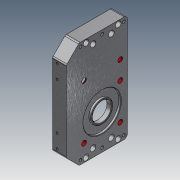
# Autodesk Inventor part: J008101
Saved by Autodesk Inventor 2018.3 (Build 223284000, 284)
## iProperties
Created: 2014-12-15
Material: ALUMINUM, 6061-T651
Vendor: HHMI: JFRC - ID&F
Document SubType Name: Modeling
Designer: ARNOLDJ
Density: 2.7 g/cm^3
Mass: 248.908 g
Surface Area: 451.626 cm^2
Volume: 92.1883 cm^3
Part Number: J008101
Description: BBP OUTER POSARM
Project: COMMON
Appearance: Polished Brushed
RuleStatus: InUse
AfterDocSave0: file://Part Number Cleaner
LAB/DEPT: COMMON
REQUESTING SCIENTIST: COMMON
SURFACE ROUGHNESS: 63 Ra
DESIGN DEPARTMENT: HHMI: JRC - ID&F
SPECIAL FINISH: ANODIZE PER MIL-A-8625F, TYPE II, CLASS 2 (BLACK)
ALTERED ITEM PART NUMBER: N/A
ALTERED ITEM VENDOR: N/A
ALTERED ITEM DESCRIPTION: N/A
Revision Number: -
Autodesk Inventor part; units mm, degrees
sketch "Sketch1" plane through (0, 0, 0) normal (0, 0, 1) x (1, 0, 0)
  line L0 (0, 127.7214) -> (0, -77.7088) projected
  line L1 (-22.86, 0) -> (3.81, 0) projected
  line L2 (-19.05, -48.3616) -> (-19.05, 98.3742)
  line L3 (0, -48.3616) -> (0, 98.3742)
  line L4 (-19.05, 98.3742) -> (0, 98.3742)
  line L5 (0, -48.3616) -> (-19.05, -48.3616)
  line L6 (-9.525, 98.3742) -> (-9.525, -48.3616) construction
  point P0 (0, 0)
  dimension "d5" = 19.05
  dimension "d67" = 0
  dimension "d149" = 48.3616
  dimension "d150" = 98.3742
  constraints: 10 end point, 2 horizontal, 2 midpoint, 1 perpendicular, 1 vertical
  measures "d5" distance between parallel lines of L2 L3
  measures "d67" distance between parallel lines of L0 L3
  measures "d149" distance between parallel lines of L5 L1
  measures "d150" distance between parallel lines of L1 L4
extrude "Extrusion1" add sketch "Sketch1" along normal blind 49.53 and the other way blind 34.925
sketch "Sketch6" plane through (0, 0, 0) normal (1, 0, 0) x (0, 1, 0)
  line L0 (0, 40.7695) -> (0, -40.1472) projected
  line L1 (-50.1548, 0) -> (123.129, 0) projected
  line L2 (-25, 25) -> (25, 25)
  line L3 (25, 25) -> (25, -25)
  line L4 (25, -25) -> (-25, -25)
  line L5 (-25, -25) -> (-25, 25)
  line L6 (0, 25) -> (0, -25) construction
  line L7 (-25, 0) -> (25, 0) construction
  point P0 (0, 0)
  point P1 (50, 25)
  point P2 (50, -25)
  dimension "d49" = 50
  dimension "d50" = 50
  dimension "d51" = 0
  dimension "d52" = 0
  dimension "d388" = 25
  constraints: 12 end point, 4 coincident, 4 midpoint, 2 parallel, 1 horizontal, 1 horizontal alignment, 1 perpendicular, 1 vertical alignment
  measures "d49" distance of L2.start L2.end
  measures "d50" distance of L4.end L2.start
  measures "d51" distance between parallel lines of L0 L6
  measures "d52" distance between parallel lines of L1 L7
  measures "d388" distance from line of L3 point (50, 25)
hole "Hole3" at (0, -25, 25) at (0, 25, -25) at (0, -25, -25) direction (-1, 0, 0) diameter 6.7564 end through all clearance for "Socket Head Cap Screw" size "M6" standard "Ansi Metric M Profile"
sketch "Sketch9" plane through (-19.05, -48.3616, 49.53) normal (-1, 0, 0) x (0, 0, 1)
  circle A0 centre (-49.53, 48.3616) radius 30 construction
  line L0 (-84.455, 146.7358) -> (-84.455, 0) projected
  line L1 (0, 0) -> (0, 146.7358) projected
  circle A1 centre (-49.53, 48.3616) radius 31.0125 construction
  line L2 (-84.455, 0) -> (0, 0) projected
  line L3 (-80.5425, 79.3741) -> (-16.0265, 79.3741)
  line L4 (-16.0265, 79.3741) -> (-16.0265, 16.5091)
  line L5 (-16.0265, 16.5091) -> (-80.5425, 16.5091)
  line L6 (-80.5425, 16.5091) -> (-80.5425, 79.3741)
  line L7 (-80.5425, 79.3741) -> (-16.0265, 79.3741)
  dimension "d80" = 60
  dimension "d87" = 62.025
  dimension "d174" = 62.865
  dimension "d231" = 64.516
  constraints: 10 end point, 2 centre point, 2 coincident, 2 horizontal, 2 parallel, 2 tangent, 1 perpendicular
  measures "d80" diameter of A0
  measures "d87" diameter of A1
  measures "d174" distance of L5.end L3.start
  measures "d231" distance between parallel lines of L4 L6
ref_plane "Work Plane1" through (-19.05, 0, 0) normal (1, 0, 0) x (0, 1, 0)
extrude "Extrusion5-Motor Cutout" cut sketch "Sketch9" against normal blind 12.7
sketch "Sketch20" plane through (-19.05, -48.3616, 49.53) normal (-1, 0, 0) x (0, 0, 1)
  line L0 (-80.5425, 16.5091) -> (-80.5425, 79.3741) projected
  line L1 (-16.0265, 16.5091) -> (-80.5425, 16.5091) projected
  line L2 (-16.0265, 79.3741) -> (-16.0265, 16.5091) projected
  line L3 (-79.2725, 129.5908) -> (-4.445, 129.5908)
  line L4 (-4.445, 129.5908) -> (-4.445, 16.5091)
  line L5 (-4.445, 16.5091) -> (-79.2725, 16.5091)
  line L6 (-79.2725, 16.5091) -> (-79.2725, 129.5908)
  line L7 (-80.5425, 79.3741) -> (-16.0265, 79.3741) projected
  line L8 (0, 0) -> (0, 146.7358) projected
  line L9 (-84.455, 146.7358) -> (-84.455, 0) projected
  line L10 (0, 146.7358) -> (-84.455, 146.7358) projected
  point P0 (-49.53, 48.3616)
  dimension "d185" = 64.516
  dimension "d232" = 4.445
  dimension "d233" = 3.9125
  dimension "d246" = 17.145
  dimension "d334" = 0
  constraints: 8 end point, 2 parallel, 1 horizontal, 1 perpendicular
  measures "d185" distance of L0.end L2.start
  measures "d232" distance between parallel lines of L8 L4
  measures "d233" distance between parallel lines of L0 L9
  measures "d246" distance between parallel lines of L10 L3
  measures "d334" distance between parallel lines of L5 L1
extrude "Extrusion12-Complete the Box cutout" cut sketch "Sketch20" against normal blind 11.43 contours L6 L7 L2 L1 | L6 L3 L4 L5 L2 L7
sketch "Sketch10" plane through (0, 0, 0) normal (1, 0, 0) x (0, 1, 0)
  circle A0 centre (0, 0) radius 13
  dimension "d93" = 26
  constraints: 1 centre point, 1 coincident
  measures "d93" diameter of A0
extrude "Extrusion6" cut sketch "Sketch10" against normal blind 25.4
sketch "Sketch25" plane through (-7.62, -48.3616, 49.53) normal (-1, 0, 0) x (0, 0, 1)
  line L0 (-4.445, 129.5908) -> (-4.445, 16.5091) projected
  line L1 (-79.2725, 129.5908) -> (-4.445, 129.5908) projected
  line L2 (-79.2725, 79.3741) -> (-79.2725, 129.5908) projected
  line L3 (-4.445, 129.5908) -> (-40.6387, 129.5908)
  line L4 (-40.6387, 84.4541) -> (-4.445, 84.4541)
  line L5 (-4.445, 84.4541) -> (-4.445, 129.5908)
  line L6 (-4.445, 129.5908) -> (-69.1125, 129.5908)
  line L7 (-69.1125, 129.5908) -> (-69.1125, 84.4541)
  line L8 (-69.1125, 84.4541) -> (-4.445, 84.4541)
  line L9 (-16.0265, 79.3741) -> (-79.2725, 79.3741) projected
  line L10 (-16.0265, 16.5091) -> (-4.445, 16.5091) projected
  line L11 (-4.445, 79.3741) -> (-13.4865, 79.3741)
  line L12 (-13.4865, 79.3741) -> (-13.4865, 16.5091)
  line L13 (-13.4865, 16.5091) -> (-4.445, 16.5091)
  line L14 (-4.445, 16.5091) -> (-4.445, 79.3741)
  point P0 (-49.53, 48.3616)
  dimension "d248" = 0
  dimension "d249" = 5.08
  dimension "d250" = 0
  dimension "d252" = 10.16
  dimension "d356" = 0
  dimension "d357" = 2.54
  constraints: 20 end point, 4 parallel, 3 horizontal, 2 perpendicular, 2 point on line
  measures "d248" distance between parallel lines of L1 L3
  measures "d249" distance between parallel lines of L4 L9
  measures "d250" distance between parallel lines of L5 L0
  measures "d252" distance between parallel lines of L7 L2
  measures "d356" distance between parallel lines of L14 L0
  measures "d357" distance from line of L9.start L12
extrude "Extrusion16" cut sketch "Sketch25" against normal blind 3.81
fillet "Fillet17" radius 3.175 7 edges at (-5.715, 36.0925, -19.5825) (-5.715, 36.0925, 45.085) (-5.715, 81.2292, -19.5825) (-5.715, 31.0125, 45.085) (-5.715, 31.0125, 36.0435) (-5.715, -31.8525, 36.0435) (-11.43, -31.8525, 45.085)
fillet "Fillet23" radius 1.651 1 edges at (-11.43, 81.2292, 45.085)
chamfer "Chamfer5" distance 17.78 angle 45 1 edges at (-9.525, -48.3616, 49.53)
chamfer "Chamfer8" distance 3.175 angle 45 2 edges at (-9.525, 98.3742, -34.925) (-9.525, -48.3616, -34.925)
chamfer "Chamfer9" distance 17.78 angle 45 1 edges at (-9.525, 98.3742, 49.53)
sketch "Sketch22" plane through (0, 0, 0) normal (1, 0, 0) x (0, 1, 0)
  point P0 (0, 0)
sketch "Sketch23" plane through (0, -31.8516, -34.925) normal (1, 0, 0) x (0, 0, -1)
  circle A0 centre (-34.925, 31.8516) radius 15.24
  circle A1 centre (-34.925, 31.8516) radius 26.035
  dimension "d221" = 52.07
  dimension "d222" = 30.48
  constraints: 2 centre point, 2 coincident
  measures "d221" diameter of A1
  measures "d222" diameter of A0
extrude "Extrusion14-rear circ cutout" cut sketch "Sketch23" against normal blind 3.175
chamfer "Chamfer10 Around rear circular cutout" distance 0.635 angle 45 3 edges at (0, 0, 26.035) (0, 0, 15.24) (0, -13, 0)
fillet "Fillet22" radius 2.413 1 edges at (-12.7, 31.0125, -31.0125)
sketch "Sketch24" plane through (-19.05, 0, 0) normal (1, 0, 0) x (0, 1, 0)
  line L0 (98.3742, 31.75) -> (98.3742, -31.75) projected
  line L1 (31.0125, -29.7425) -> (81.2292, -29.7425) projected
  line L2 (62.6618, -29.7425) -> (27.7368, -29.7425)
  line L3 (27.7368, -29.7425) -> (27.7368, -31.6475)
  line L4 (27.7368, -31.6475) -> (62.6618, -31.6475)
  line L5 (62.6618, -31.6475) -> (62.6618, -29.7425)
  point P0 (0, 0)
  point P1 (106.426, 30.4349)
  point P2 (106.426, -30.4349)
  point P3 (-28.6775, -31.0125)
  point P4 (91.3375, -31.0125)
  point P5 (98.3742, -34.925)
  point P6 (106.426, -31.75)
  point P7 (106.426, 31.75)
  point P8 (-32.4875, -31.0125)
  point P9 (81.2292, -29.7425)
  point P10 (98.3742, 49.53)
  point P11 (-32.4875, -29.7425)
  point P12 (98.3742, -31.75)
  dimension "d239" = 1.905
  dimension "d240" = 70.6374
  dimension "d241" = 34.925
  dimension "d242" = 0
  constraints: 8 end point, 2 parallel, 1 horizontal, 1 perpendicular, 2 other
  measures "d241" distance of L3.end L4.end
  measures "d242" vertical extent of L2
extrude "Extrusion15" cut sketch "Sketch24" along normal blind 7.62
fillet "Fillet15" radius 2.413 2 edges at (-15.24, 62.6618, -31.6475) (-15.24, 27.7368, -31.6475)
fillet "Fillet16" radius 2.413 4 edges at (-13.335, 81.2292, -29.7425) (-6.985, 31.0125, 33.5035) (-6.985, -31.8525, 33.5035) (-12.7, -31.8525, -31.0125)
sketch "Sketch29" plane through (-19.05, 0, 0) normal (1, 0, 0) x (0, 1, 0)
  line L0 (84.8551, 23.9395) -> (89.6429, 23.9395)
  line L1 (89.6429, 23.9395) -> (89.6429, 29.4005)
  line L2 (89.6429, 29.4005) -> (84.8551, 29.4005)
  line L3 (84.8551, 29.4005) -> (84.8551, 23.9395)
  line L4 (84.8551, 23.9395) -> (89.6429, 29.4005) construction
  line L5 (89.6429, 23.9395) -> (84.8551, 29.4005) construction
  line L6 (98.3742, 31.75) -> (98.3742, -31.75) projected
  point P0 (0, 0)
  point P1 (87.249, -26.67)
  point P2 (87.249, 26.67)
  dimension "d296" = 53.34
  dimension "d297" = 26.67
  dimension "d298" = 87.249
  dimension "d299" = 4.7879
  dimension "d300" = 5.461
  dimension "d311" = 11.1252
  constraints: 12 end point, 2 midpoint, 2 parallel, 1 horizontal, 1 perpendicular, 1 vertical alignment
  measures "d296" distance of point (87.249, 26.67) point (87.249, -26.67)
  measures "d297" vertical distance of point (0, 0) point (87.249, 26.67)
  measures "d298" horizontal distance of point (0, 0) point (87.249, 26.67)
  measures "d299" distance of L1.end L2.end
  measures "d300" distance of L0.end L1.end
  measures "d311" distance from line of point (87.249, 26.67) L6
extrude "Extrusion19" cut sketch "Sketch29" along normal blind 10.16
hole "Hole11" at (-19.05, 87.249, -26.67) direction (1, 0, 0) diameter 4.7879 depth 10.16 tip angle 118
fillet "Fillet19" radius 1.905 4 edges at (-13.97, 89.6429, 29.4005) (-13.97, 84.8551, 29.4005) (-13.97, 84.8551, 23.9395) (-13.97, 89.6429, 23.9395)
sketch "Sketch30" plane through (0, 0, 0) normal (1, 0, 0) x (0, 1, 0)
  line L0 (93.599, 22.225) -> (93.599, -22.225) construction
  line L1 (93.599, 0) -> (87.121, 0) construction
  circle A0 centre (87.249, -26.67) radius 2.3939 construction
  point P0 (0, 0)
  point P1 (87.249, -12.7)
  point P2 (87.249, 12.7)
  dimension "d312" = 44.45
  dimension "d313" = 25.4
  dimension "d314" = 12.7
  dimension "d315" = 0
  dimension "d316" = 0
  dimension "d317" = 6.35
  dimension "d387" = 6.35
  constraints: 4 end point, 2 vertical alignment, 1 horizontal, 1 midpoint, 1 vertical
  measures "d312" distance of L0.end L0.start
  measures "d313" distance of point (87.249, -12.7) point (87.249, 12.7)
  measures "d314" distance from line of L1 point (87.249, 12.7)
  measures "d315" distance from line of L1 point (0, 0)
  measures "d316" horizontal distance of point (87.249, -12.7) A0.centre
  measures "d317" horizontal distance of L0.end A0.centre
  measures "d387" horizontal distance of L0.start point (87.249, 12.7)
hole "Hole12" at (0, 93.599, 22.225) at (0, 87.249, 12.7) at (0, 87.249, -12.7) at (0, 93.599, -22.225) direction (-1, 0, 0) diameter 4.4958 end through all counterbore diameter 8.001 counterbore depth 7.62 clearance for "Socket Head Cap Screw" size "M4" standard "Ansi Metric M Profile"
sketch "Sketch31" plane through (-19.05, 0, 0) normal (1, 0, 0) x (0, 1, 0)
  line L0 (81.2292, -27.3295) -> (81.2292, 43.434) projected
  line L1 (95.8342, 17.145) -> (95.8342, -17.145)
  circle A0 centre (87.249, 12.7) radius 2.2479 projected
  circle A1 centre (93.599, 22.225) radius 2.2479 projected
  circle A2 centre (87.249, -12.7) radius 2.2479 projected
  circle A3 centre (93.599, -22.225) radius 2.2479 projected
  line L2 (98.3742, 31.75) -> (98.3742, -31.75) construction
  line L3 (84.4042, 0) -> (95.8342, 0) construction
  circle A4 centre (87.249, -12.7) radius 5.08 construction
  circle A5 centre (93.599, 22.225) radius 5.08 construction
  circle A6 centre (87.249, 12.7) radius 2.2479 construction
  circle A7 centre (87.249, 12.7) radius 5.08 construction
  circle A8 centre (93.599, -22.225) radius 5.08 construction
  line L4 (95.8342, 17.145) -> (92.329, 17.145)
  line L5 (92.329, 17.145) -> (92.329, 7.62)
  line L6 (92.329, 7.62) -> (83.7692, 7.62)
  line L7 (83.7692, 7.62) -> (83.7692, -7.62)
  line L8 (83.7692, -7.62) -> (92.329, -7.62)
  line L9 (92.329, -7.62) -> (92.329, -17.145)
  line L10 (92.329, -17.145) -> (95.8342, -17.145)
  point P0 (0, 0)
  point P1 (81.8642, 42.672)
  point P2 (81.2292, 45.085)
  point P3 (81.2292, 41.91)
  dimension "d326" = 2.54
  dimension "d329" = 0
  dimension "d358" = 10.16
  dimension "d359" = 34.29
  dimension "d360" = 3.5052
  dimension "d361" = 2.54
  constraints: 18 end point, 5 perpendicular, 4 centre point, 4 coincident, 3 equal radius, 2 horizontal, 2 point on line, 1 midpoint, 1 tangent, 1 vertical, 1 other
  measures "d326" distance between parallel lines of L2 L1
  measures "d329" distance from line of point (0, 0) L3
  measures "d358" diameter of A4
  measures "d359" distance of L1.start L1.end
  measures "d360" distance of L1.start L4.end
extrude "Extrusion20" cut sketch "Sketch31" along normal blind 12.7 contours L1 L10 L9 L8 L7 L6 L5 L4
fillet "Fillet20" radius 1.651 6 edges at (-12.7, 95.8342, 17.145) (-12.7, 95.8342, -17.145) (-12.7, 83.7692, -7.62) (-12.7, 83.7692, 7.62) (-12.7, 92.329, 17.145) (-12.7, 92.329, -17.145)
fillet "Fillet25" radius 4.445 2 edges at (-12.7, 92.329, -7.62) (-12.7, 92.329, 7.62)
ref_plane "Work Plane2-Midplane of part" through (-19.05, 25.0063, 31.75) normal (0, -1, 0) x (1, 0, 0)
fillet "Fillet21" radius 3.175 8 edges at (-9.525, 98.3742, 31.75) (-9.525, 98.3742, -31.75) (-9.525, 95.1992, -34.925) (-9.525, -45.1866, -34.925) (-9.525, 80.5942, 49.53) (-9.525, -30.5816, 49.53) (-9.525, -48.3616, 31.75) (-9.525, -48.3616, -31.75)
sketch "Sketch32" plane through (0, 0, 0) normal (1, 0, 0) x (0, 1, 0)
  line L0 (0, 66.421) -> (0, -51.816) projected
  line L1 (-77.7088, 0) -> (127.7214, 0) projected
  line L2 (98.3742, -30.4349) -> (98.3742, 30.4349) projected
  circle A0 centre (92.9132, -29.845) radius 2.9972 construction
  circle A1 centre (92.9132, -29.845) radius 8 construction
  line L3 (-43.8715, -34.925) -> (93.8841, -34.925) projected
  point P0 (0, 0)
  point P1 (92.9132, 29.845)
  point P2 (92.9132, 0)
  dimension "d338" = 5.461
  dimension "d339" = 5.9944
  dimension "d340" = 16
  dimension "d341" = 2.4638
  dimension "d343" = 29.845
  dimension "d344" = 5.08
  dimension "d345" = 29.845
  dimension "d346" = 5.461
  constraints: 2 centre point, 2 coincident, 1 point on line, 1 vertical alignment
  measures "d338" distance from line of point (92.913, -29.845) L2
  measures "d339" diameter of A0
  measures "d340" diameter of A1
  measures "d341" distance edge to line of A0 L2
  measures "d343" distance from line of A0.centre L1
  measures "d344" distance from line of L3 A0.centre
  measures "d345" distance from line of L1 point (92.913, 29.845)
  measures "d346" distance from line of L2 point (92.913, 29.845)
hole "Hole13" at (0, 92.9132, 29.845) at (0, 92.9132, -29.845) at (0, 92.9132, 0) direction (-1, 0, 0) diameter 4.1402 depth 14.1986 tip angle 118
sketch "Sketch34" plane through (0, 0, -34.925) normal (0, 0, -1) x (-1, 0, 0)
  line L0 (12.7, 76.1492) -> (12.7, 57.0992) construction
  line L1 (19.05, 98.3742) -> (0, 98.3742) projected
  line L2 (19.05, 93.8841) -> (19.05, -43.8715) projected
  line L3 (12.7, 57.0992) -> (12.7, -26.1366) construction
  line L4 (0, -48.3616) -> (19.05, -48.3616) construction
  point P0 (0, 0)
  point P1 (12.7, -7.0866)
  dimension "d375" = 19.05
  dimension "d376" = 6.35
  dimension "d377" = 22.225
  dimension "d385" = 22.225
  dimension "d386" = 19.05
  constraints: 4 end point, 3 coincident, 2 vertical, 1 point on line
  measures "d375" distance of L0.start L0.end
  measures "d376" distance between parallel lines of L2 L0
  measures "d377" distance from line of point (12.7, 76.149) L1
  measures "d385" distance from line of L3.end L4
  measures "d386" distance of point (12.7, -26.137) point (12.7, -7.087)
hole "Hole15" at (-12.7, 76.1492, -34.925) at (-12.7, 57.0992, -34.925) at (-12.7, -7.0866, -34.925) at (-12.7, -26.1366, -34.925) direction (0, 0, 1) diameter 3.2512 end through all
ref_plane "Work Plane3" through (-11.43, 31.0125, -29.7425) normal (0, 0, 1) x (1, 0, 0)
mirror "Mirror1" about plane through (-19.05, 25.0063, 31.75) normal (0, -1, 0) of "Extrusion20", "Hole12", "Fillet19", "Hole11", "Extrusion19", "Hole13", "Fillet25", "Fillet20"
sketch "Sketch35" plane through (-3.81, -48.3616, 49.53) normal (-1, 0, 0) x (0, 0, 1)
  point P0 (-49.53, 48.3616)
  point P1 (-24.53, 98.3616)
hole "Hole16" at (-3.81, 50, 25) direction (1, 0, 0) diameter 6.604 end through all countersink diameter 12.5984 countersink angle 90 clearance for "Flat Head Machine Screw" size "M6" standard "Ansi Metric M Profile"
sketch "Sketch36" plane through (-7.62, -48.3616, 49.53) normal (-1, 0, 0) x (0, 0, 1)
  point P0 (-49.53, 48.3616)
  point P1 (-74.53, 98.3616)
hole "Hole17" at (-7.62, 50, -25) direction (1, 0, 0) diameter 6.7564 end through all counterbore diameter 11.1125 counterbore depth 5.9944 clearance for "Socket Head Cap Screw" size "M6" standard "Ansi Metric M Profile"
fillet "Fillet26" radius 1.524 2 edges at (-5.715, 48.7661, -19.5825) (-5.715, 51.2339, -19.5825)
sketch "Sketch37" plane through (-7.62, -48.3616, 49.53) normal (-1, 0, 0) x (0, 0, 1)
  circle A0 centre (-74.53, 98.3616) radius 5.5562 projected
  circle A1 centre (-74.53, 98.3616) radius 3.3782 projected
  circle A2 centre (-74.53, 98.3616) radius 5.5563
  point P0 (-49.53, 48.3616)
  constraints: 1 centre point, 1 coincident, 1 concentric
extrude "Extrusion21" cut sketch "Sketch37" along normal up to next
body "Solid1"
